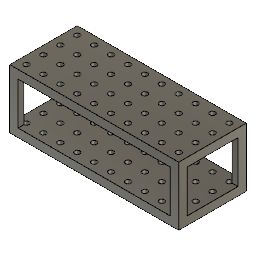
tube test rack v4 (Autodesk Fusion 360 design; units mm, degrees)
Autodesk Fusion 360 part; units mm, degrees
sketch "base" plane through (0, 0, 0) normal (0, 0, 1) x (1, 0, 0)
  line L0 (-100, 40) -> (0, 40)
  line L1 (0, 40) -> (0, 0)
  line L2 (0, 0) -> (-100, 0)
  line L3 (-100, 0) -> (-100, 40)
  dimension "d1" = 40
  dimension "d2" = 100
  constraint horizontal L0
  constraint vertical L1
  constraint horizontal L2
  constraint vertical L3
  constraint coincident L1.end L2.start
  measures "d1" distance of L0.end L1.end
  measures "d2" distance of L0.start L0.end
extrude "Extrude1" add sketch "base" along normal blind 5
sketch "stands" plane through (0, 0, 5) normal (0, 0, 1) x (-1, 0, 0)
  line L0 (100, 0) -> (0, 0)
  line L1 (0, 0) -> (0, -40)
  line L2 (0, -40) -> (100, -40)
  line L3 (100, -40) -> (100, 0)
  line L4 (100, -40) -> (95, -40)
  line L5 (95, -40) -> (95, -35)
  line L6 (95, -35) -> (100, -35)
  line L7 (100, -35) -> (100, -40)
  line L8 (5, -35) -> (5, -40)
  line L9 (5, -40) -> (0, -40)
  line L10 (0, -40) -> (0, -35)
  line L11 (0, -35) -> (5, -35)
  line L12 (100, 0) -> (100, -5)
  line L13 (100, -5) -> (95, -5)
  line L14 (95, -5) -> (95, 0)
  line L15 (95, 0) -> (100, 0)
  line L16 (5, 0) -> (5, -5)
  line L17 (5, -5) -> (0, -5)
  line L18 (0, -5) -> (0, 0)
  line L19 (0, 0) -> (5, 0)
  dimension "d6" = 5
  dimension "d7" = 5
  dimension "d8" = 5
  dimension "d11" = -95
  dimension "d12" = 35
  dimension "d13" = 90
  dimension "d14" = 30
  constraint coincident L2.end L3.start
  constraint horizontal L4
  constraint vertical L7
  measures "d6" distance of L2.end L4.end
  measures "d7" distance of L4.end L5.end
  measures "d8" distance of L4 L6
  measures "d13" distance of L4.end L8.end
  measures "d14" distance of L6.end L12.end
extrude "Extrude2" add sketch "stands" along normal blind 25 contours L0 L3 L12 L13 L14 L15 | L0 L1 L16 L17 L18 L19 | L2 L3 L4 L5 L6 L7 | L1 L2 L8 L9 L10 L11
sketch "top" plane through (0, 0, 30) normal (0, 0, 1) x (-1, 0, 0)
  line L0 (95, 0) -> (95, -5)
  line L1 (95, -5) -> (100, -5)
  line L2 (100, -5) -> (100, 0)
  line L3 (100, 0) -> (95, 0)
  line L4 (100, -40) -> (0, -40)
  line L5 (0, -40) -> (0, 0)
  line L6 (0, 0) -> (100, 0)
  line L7 (100, 0) -> (100, -40)
  point P0 (100, -40)
  constraint horizontal L4
  constraint vertical L5
  constraint horizontal L6
  constraint vertical L7
  constraint coincident L5.end L6.start
  constraint coincident P0 L4.start
extrude "Extrude3" add sketch "top" along normal blind 5
sketch "tube holes" plane through (0, 0, 35) normal (0, 0, 1) x (-1, 0, 0)
  line L0 (100, 0) -> (0, 0)
  line L1 (0, 0) -> (0, -40)
  line L2 (0, -40) -> (100, -40)
  line L3 (100, -40) -> (100, 0)
  circle A0 centre (95, -35) radius 1.55
  circle A1 centre (85, -35) radius 1.55
  circle A2 centre (75, -35) radius 1.55
  circle A3 centre (65, -35) radius 1.55
  circle A4 centre (55, -35) radius 1.55
  circle A5 centre (45, -35) radius 1.55
  circle A6 centre (35, -35) radius 1.55
  circle A7 centre (25, -35) radius 1.55
  circle A8 centre (15, -35) radius 1.55
  circle A9 centre (5, -35) radius 1.55
  circle A10 centre (95, -25) radius 1.55
  circle A11 centre (85, -25) radius 1.55
  circle A12 centre (75, -25) radius 1.55
  circle A13 centre (65, -25) radius 1.55
  circle A14 centre (55, -25) radius 1.55
  circle A15 centre (45, -25) radius 1.55
  circle A16 centre (35, -25) radius 1.55
  circle A17 centre (25, -25) radius 1.55
  circle A18 centre (15, -25) radius 1.55
  circle A19 centre (5, -25) radius 1.55
  circle A20 centre (95, -15) radius 1.55
  circle A21 centre (85, -15) radius 1.55
  circle A22 centre (75, -15) radius 1.55
  circle A23 centre (65, -15) radius 1.55
  circle A24 centre (55, -15) radius 1.55
  circle A25 centre (45, -15) radius 1.55
  circle A26 centre (35, -15) radius 1.55
  circle A27 centre (25, -15) radius 1.55
  circle A28 centre (15, -15) radius 1.55
  circle A29 centre (5, -15) radius 1.55
  circle A30 centre (95, -5) radius 1.55
  circle A31 centre (85, -5) radius 1.55
  circle A32 centre (75, -5) radius 1.55
  circle A33 centre (65, -5) radius 1.55
  circle A34 centre (55, -5) radius 1.55
  circle A35 centre (45, -5) radius 1.55
  circle A36 centre (35, -5) radius 1.55
  circle A37 centre (25, -5) radius 1.55
  circle A38 centre (15, -5) radius 1.55
  circle A39 centre (5, -5) radius 1.55
  point P0 (95, -35)
  dimension "d19" = 3.1
  dimension "d22" = -10
  dimension "d23" = 10
  constraint coincident P0 A0.centre
  measures "d19" diameter of A0
extrude "Extrude4" cut sketch "tube holes" against normal blind 34 contours A0 | A1 | A2 | A3 | A4 | A5 | A6 | A7 | A8 | A9 | A10 | A11 | A12 | A13 | A14 | A15 | A16 | A17 | A18 | A19 | A20 | A21 | A22 | A23 | A24 | A25 | A26 | A27 | A28 | A29 | A30 | A31 | A32 | A33 | A34 | A35 | A36 | A37 | A38 | A39
hole "Hole1" [rolled back] hole depth 30 hole diameter 2.4 tip angle 118 csdiameter 3.41 csangle 90
